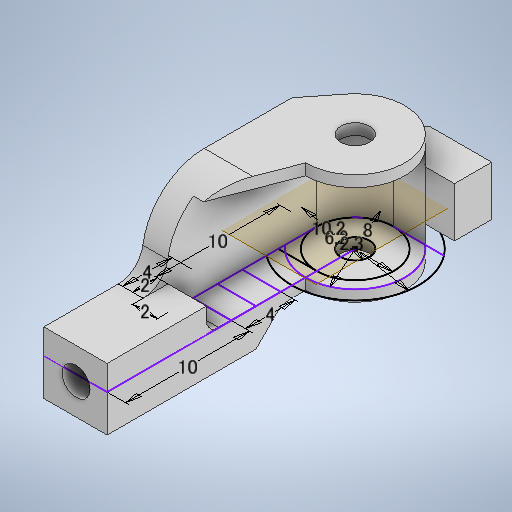
# Autodesk Inventor part: srod2.7_2.25
Saved by Autodesk Inventor 2025 (Build 290162000, 162)
## iProperties
Created: 2024-08-08
Part Number: srod2.7_2.25
Material: 一般
Document SubType Name: Modeling
Designer: Saigusa
Density: 1 g/cm^3
Appearance: 既定
Author: Saigusa
Autodesk Inventor part; units mm, degrees
ref_plane "YZ Plane" through (0, 0, 0) normal (1, 0, 0) x (0, 1, 0)
ref_plane "XZ Plane" through (0, 0, 0) normal (0, 1, 0) x (-1, 0, 0)
ref_plane "XY Plane" through (0, 0, 0) normal (0, 0, 1) x (1, 0, 0)
sketch "スケッチ1" plane through (0, 0, 0) normal (0, 1, 0) x (-1, 0, 0)
  circle A0 centre (0, 0) radius 1.15
  circle A1 centre (0, 0) radius 3.1
  circle A2 centre (0, 0) radius 5.1
  line L0 (3.1, 0) -> (5.1, 0)
  line L1 (5.1, 0) -> (5.1, 10)
  line L2 (5.1, 10) -> (3.1, 10)
  line L3 (3.1, 10) -> (3.1, 0)
  line L4 (0, 3.1) -> (3.1, 3.1)
  line L5 (5.1, 0) -> (1.8843, -2.4616)
  line L6 (5.1, 10) -> (0, 10)
  line L7 (0, 10) -> (0, 20)
  line L8 (0, 20) -> (5.1, 20)
  line L9 (5.1, 20) -> (5.1, 10)
  line L10 (0, 10) -> (0, 0)
  line L11 (0, -3.1) -> (-4.0497, -3.1)
  line L12 (3.1, 10) -> (5.1, 10)
  line L13 (5.1, 10) -> (5.1, 12)
  line L14 (5.1, 12) -> (3.1, 12)
  line L15 (3.1, 12) -> (3.1, 10)
  line L16 (3.1, 12) -> (0, 12)
  line L17 (0, 12) -> (0, 10)
  line L18 (0, 10) -> (3.1, 10)
  line L19 (3.1, 10) -> (3.1, 12)
  line L20 (0, 12) -> (5.1, 12)
  line L21 (5.1, 12) -> (5.1, 8)
  line L22 (5.1, 8) -> (0, 8)
  line L23 (0, 8) -> (0, 12)
  circle A3 centre (0, 0) radius 4
  line L24 (5.1, 0) -> (3.1373, -2.4815)
  line L25 (5.1, 10) -> (0, 10)
  line L26 (0, 10) -> (0, 6)
  line L27 (0, 6) -> (5.1, 6)
  line L28 (5.1, 6) -> (5.1, 10)
  point P0 (0, 5.1)
  point P1 (-2.5278, -3.1)
  point P2 (0, 4)
  dimension "d2" = 10.2
  dimension "d37" = 8
  dimension "d0" = 2.3
  dimension "d1" = 6.2
  dimension "d3" = 10
  dimension "d4" = 10
  dimension "d7" = 2
  dimension "d8" = 2
  dimension "d22" = 4
  dimension "d42" = 4
  constraints: 58 end point, 12 parallel, 8 perpendicular, 6 horizontal, 4 coincident, 4 point on circle, 4 point on line, 2 centre point, 2 tangent, 1 vertical, 7 other
  measures "d0" diameter of A0
  measures "d1" diameter of A1
  measures "d3" distance of L1.end L0.end
  measures "d4" distance of L6.end L7.end
  measures "d7" distance of L14.end L13.end
  measures "d8" distance of L13.end L12.end
  measures "d22" distance of L20.end L21.end
  measures "d42" distance of L26.end L25.end
extrude "押し出し1" add sketch "スケッチ1" along normal blind 7.1 contours L0 A3 L5 A1 | L3 A3 L0 | L5 A3 L11 A1 | A3 L3 A2 L0 | L0 L5 A3 | L5 L24 A3 | A2 L3 L27 L1 | L27 L3 L22 L1 | L22 L3 L2 L1 | L2 L15 L14 L9
extrude "押し出し2" add sketch "スケッチ1" against normal blind 0.9 contours A1 | L0 A3 L5 A1 | L3 A3 L0 | A1 L4 A3 L3 | L10 A3 L4 | A1 L11 A3 L10 | L5 A3 L11 A1 | A3 L3 A2 L0 | L0 L5 A3 | A3 L4 L3 | A3 L10 A2 L3 L4 | L5 L24 A3 | A2 L3 L27 L1 | L10 L27 L3 A2 | L27 L3 L22 L1 | L10 L22 L3 L27 | L22 L3 L2 L1 | L10 L6 L3 L22 | L2 L15 L14 L9 | L7 L16 L15 L6 | L14 L16 L7 L8 L9
sketch "スケッチ2" plane through (0, 7.1, 0) normal (0, 1, 0) x (1, 0, 0)
  circle A0 centre (0, 0) radius 1.15
  circle A1 centre (0, 0) radius 3.1
  circle A2 centre (0, 0) radius 5.1
  line L0 (0, -12) -> (-5.1, -12)
  line L1 (0, 0) -> (-5.1, 0)
  line L2 (-5.1, 0) -> (-5.1, -12)
  line L3 (-5.1, -12) -> (0, -12)
  line L4 (0, -12) -> (0, 0)
  line L5 (-5.1, 0) -> (-1.8843, 2.4616)
  line L6 (-5.1, 0) -> (-1.8843, 2.4616)
  circle A3 centre (0, 0) radius 4
  line L7 (-5.1, 0) -> (-3.1373, 2.4815) projected
  line L8 (-5.1, 0) -> (-3.1373, 2.4815)
  line L9 (0, -4) -> (-3.1639, -4)
  line L10 (-3.1, -12) -> (-3.1, 0) projected
  line L11 (0, -4) -> (-3.1, -12)
  point P0 (0, -5.1)
  point P1 (0, -3.1)
  point P2 (0, -4)
  dimension "d13" = 10.2
  dimension "d11" = 2.3
  dimension "d12" = 6.2
  dimension "d14" = 5.1
  dimension "d15" = 12
  dimension "d38" = 8
  constraints: 20 end point, 4 coincident, 3 centre point, 3 equal length, 2 perpendicular, 2 point on circle, 2 tangent, 1 horizontal, 1 point on line, 3 other
  measures "d11" diameter of A0
  measures "d12" diameter of A1
  measures "d14" distance of L3.end L0.end
  measures "d15" distance of L0.end L1.end
  measures "d38" diameter of A3
extrude "押し出し3" add sketch "スケッチ2" along normal blind 0.9 contours A0 L1 A1 L4 | A0 L4 A1 L1 | L1 A3 L5 A1 | L10 A3 L1 | A1 L4 A3 L10 | A1 L5 A3 L4 | A3 L10 L9 A2 L1 | L1 L5 A3 | A3 L9 L10 | L11 A2 L10 L9 | L5 L7 A3 | A2 L10 L0 L2 | L10 A2 L9 | L11 L10 A2
extrude "押し出し4" add sketch "スケッチ1" along normal blind 2 contours L14 L16 L7 L8 L9
extrude "押し出し5" add sketch "スケッチ1" against normal blind 3 contours L27 L3 L22 L1 | L10 L22 L3 L27 | L22 L3 L2 L1 | L10 L6 L3 L22 | L2 L15 L14 L9 | L7 L16 L15 L6 | L14 L16 L7 L8 L9
sketch "スケッチ3" plane through (-5.1, 2, 20) normal (0, 0, 1) x (1, 0, 0)
  line L0 (0, -5) -> (0, 0) projected
  line L1 (0, 0) -> (2.6, 0)
  line L2 (2.6, 0) -> (2.6, -2.5)
  line L3 (2.6, -2.5) -> (0, -2.5)
  line L4 (0, -2.5) -> (0, 0)
  circle A0 centre (2.6, -2.5) radius 1.125
  point P0 (5.1, -2)
  dimension "d26" = 2.6
  dimension "d27" = 2.5
  dimension "d28" = 2.25
  constraints: 8 end point, 2 parallel, 1 centre point, 1 coincident, 1 horizontal, 1 perpendicular
  measures "d26" distance of L2.end L3.end
  measures "d27" distance of L1.end L2.end
  measures "d28" diameter of A0
hole "穴1" at (-2.5, -0.5, 20) direction (0, 0, -1) diameter 2.25 depth 7
fillet "フィレット1" radius 2 1 edges at (-4.1, 2, 12)
fillet "フィレット2" radius 1 1 edges at (-1.55, 0, 12)
fillet "フィレット4" radius 5 1 edges at (-4.1, 8, 12)
chamfer "面取り2" distance 2 angle 45 1 edges at (-2.55, -3, 6)
fillet "フィレット5" radius 5 1 edges at (-2.55, -0.9, 6)
ref_plane "作業平面1" through (0, 3.55, 0) normal (0, 1, 0) x (1, 0, 0)
sketch "スケッチ4" plane through (0, 3.55, 0) normal (0, 1, 0) x (1, 0, 0)
  circle A0 centre (0, 0) radius 5
  circle A1 centre (0, 0) radius 3
  arc A2 (0, -4) -> (-3.1373, 2.4815) centre (0, 0) ccw projected
  line L0 (0, 0) -> (0, 3)
  line L1 (0, 3) -> (5, 3)
  line L2 (0, 3) -> (5, 3) construction
  line L3 (5, 3) -> (5, 6)
  line L4 (5, 6) -> (0, 6)
  line L5 (0, 6) -> (-2.9814, 2.6667)
  point P0 (2.6458, 3)
  dimension "d49" = 6
  dimension "d48" = 10
  dimension "d50" = 5
  dimension "d51" = 0
  dimension "d52" = 3
  constraints: 12 end point, 3 horizontal, 2 coincident, 2 perpendicular, 1 centre point, 1 collinear, 1 point on circle, 1 tangent, 1 vertical alignment, 2 other
  measures "d48" diameter of A0
  measures "d50" distance of L0.end L1.end
  measures "d51" distance between parallel lines of L1 L2
  measures "d52" distance of L2.end L3.end
extrude "押し出し6" add sketch "スケッチ4" along normal mid plane 4 contours L1 A2 L5 A0 | A0 L5 L4 L3 L1 picked at (3.2919, 3.2722)
